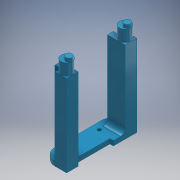
# Autodesk Inventor part: blue_part-july21
Saved by Autodesk Inventor 2017 SP1 (Build 210196100, 196)
## iProperties
Created: 2016-07-25
Part Number: blue_part-july21
Material: Plastique ABS
Document SubType Name: Modeling
Designer: tmonglon
Density: 1.06 g/cm^3
Appearance: Bleu ciel foncé
Author: tmonglon
Autodesk Inventor part; units mm, degrees
ref_plane "YZ Plane" through (0, 0, 0) normal (1, 0, 0) x (0, 1, 0)
ref_plane "XZ Plane" through (0, 0, 0) normal (0, 1, 0) x (-1, 0, 0)
ref_plane "XY Plane" through (0, 0, 0) normal (0, 0, 1) x (1, 0, 0)
sketch "Esquisse1" plane through (0, 0, 0) normal (0, 0, 1) x (1, 0, 0)
  line L0 (0, 0) -> (-10, 0)
  line L1 (-10, 0) -> (-10, 30)
  line L2 (-10, 30) -> (0, 30)
  line L3 (0, 0) -> (-5, 0)
  line L4 (-5, 0) -> (-5, 5)
  line L5 (-5, 5) -> (0, 5)
  line L6 (0, 5) -> (0, 0)
  line L7 (0, 4) -> (-3, 4)
  line L8 (-3, 4) -> (-3, 1)
  line L9 (-3, 1) -> (0, 1)
  line L10 (0, 1) -> (0, 4)
  line L11 (-1.5, 5) -> (-1.5, 20)
  line L12 (-1.5, 20) -> (0, 20)
  line L13 (0, 30) -> (0, 20)
  line L14 (0, 5) -> (0, 0)
  line L15 (0, 29) -> (-3, 29)
  line L16 (-3, 29) -> (-3, 26)
  line L17 (-3, 26) -> (0, 26)
  line L18 (0, 26) -> (0, 29)
  line L19 (0, 25) -> (-5, 25)
  line L20 (-5, 25) -> (-5, 30)
  line L21 (-5, 25) -> (-7.5, 25)
  line L22 (-7.5, 25) -> (-7.5, 27.5)
  line L23 (-7.5, 27.5) -> (-5, 27.5)
  line L24 (-5, 27.5) -> (-5, 25)
  line L25 (-5, 0) -> (-7.5, 0)
  line L26 (-5, 2.5) -> (-5, 0)
  line L27 (-5, 5) -> (-7.5, 5)
  line L28 (-7.5, 5) -> (-7.5, 2.5)
  line L29 (-7.5, 2.5) -> (-5, 2.5)
  line L30 (-5, 2.5) -> (-5, 5)
  line L31 (-3, 26) -> (0, 26)
  line L32 (0, 26) -> (0, 29)
  line L33 (0, 29) -> (-3, 29)
  line L34 (-3, 29) -> (-3, 26)
  line L35 (-3, 1) -> (0, 1)
  line L36 (0, 1) -> (0, 4)
  line L37 (0, 4) -> (-3, 4)
  line L38 (-3, 4) -> (-3, 1)
  dimension "d0" = 10
  dimension "d1" = 30
  dimension "d2" = 5
  dimension "d3" = 5
  dimension "d4" = 3
  dimension "d5" = 3
  dimension "d6" = 1
  dimension "d7" = 15
  dimension "d9" = 3
  dimension "d10" = 3
  dimension "d11" = 1
  dimension "d12" = 5
  dimension "d13" = 5
  dimension "d14" = 2.5
  dimension "d15" = 2.5
  dimension "d20" = 2.5
  dimension "d21" = 2.5
  constraints: 78 end point, 17 parallel, 11 perpendicular, 10 horizontal, 3 point on line, 2 midpoint, 1 vertical
  measures "d0" distance of L0.start L0.end
  measures "d1" distance of L2.end L0.start
  measures "d2" distance of L4.end L5.end
  measures "d3" distance of L3.end L4.end
  measures "d4" distance of L8.end L9.end
  measures "d5" distance of L7.end L8.end
  measures "d6" distance between parallel lines of L5 L7
  measures "d7" distance of L11.start L11.end
  measures "d9" distance of L15.end L16.end
  measures "d10" distance of L16.end L17.end
  measures "d11" distance between parallel lines of L2 L15
  measures "d12" distance of L19.start L19.end
  measures "d13" distance of L19.end L20.end
  measures "d14" distance of L22.end L23.end
  measures "d15" distance of L21.end L22.end
  measures "d20" distance of L28.end L29.end
  measures "d21" distance of L27.end L28.end
extrude "Extrusion1" add sketch "Esquisse1" along normal blind 41.5 contours L0 L4 L5 L6 L7 L8 L9 | L9 L8 L7 L6 | L2 L13 L15 L16 L17 L19 L20 | L13 L17 L16 L15
extrude "Extrusion2" add sketch "Esquisse1" along normal blind 35 contours L29 L28 L27 L4 | L20 L21 L22 L23
extrude "Extrusion4" add sketch "Esquisse1" along normal blind 2 contours L0 L1 L2 L20 L23 L22 L21 L19 L13 L12 L11 L5 L27 L28 L29 L4
fillet "Congé1" radius 5 2 edges at (-10, 0, 1) (-10, 30, 1)
sketch "Esquisse3" plane through (0, 0, 0) normal (0, 0, -1) x (-1, 0, 0)
  circle A0 centre (7, 9) radius 0.7
  circle A1 centre (7, 21) radius 0.7
  line L0 (0, 0) -> (0, 5) projected
  line L1 (0, 20) -> (0, 30) projected
  line L2 (5, 0) -> (0, 0) projected
  dimension "d29" = 1.4
  dimension "d30" = 1.4
  dimension "d31" = 12
  dimension "d32" = 7
  dimension "d33" = 7
  dimension "d34" = 9
  constraints: 2 centre point
  measures "d29" diameter of A0
  measures "d30" diameter of A1
  measures "d31" distance of A1.centre A0.centre
  measures "d32" distance from line of L0 A0.centre
  measures "d33" distance from line of L1 A1.centre
  measures "d34" distance from line of L2 A0.centre
extrude "Extrusion5" cut sketch "Esquisse3" against normal through all
fillet "Congé2" radius 2 2 edges at (-3.75, 25, 2) (-4.5, 5, 2)
sketch "Esquisse8" plane through (0, 0, 41.5) normal (0, 0, 1) x (1, 0, 0)
  line L0 (0, 0) -> (0, 5) projected
  line L1 (0, 5) -> (-5, 5) projected
  line L2 (-5, 5) -> (-5, 0) projected
  line L3 (-5, 0) -> (0, 0) projected
  line L4 (0, 30) -> (-5, 30) projected
  line L5 (-5, 30) -> (-5, 25) projected
  line L6 (-5, 25) -> (0, 25) projected
  line L7 (0, 25) -> (0, 30) projected
  circle A0 centre (-2.5, 2.5) radius 2.4
  circle A1 centre (-2.5, 27.5) radius 2.4
  dimension "d42" = 4.8
  dimension "d43" = 2.5
  dimension "d44" = 2.5
  dimension "d45" = 4.8
  dimension "d48" = 2.5
  dimension "d49" = 2.5
  constraints: 2 centre point
  measures "d42" diameter of A0
  measures "d43" distance from line of L7 A1.centre
  measures "d44" distance from line of L4 A1.centre
  measures "d45" diameter of A1
  measures "d48" distance from line of L0 A0.centre
  measures "d49" distance from line of L3 A0.centre
extrude "Extrusion8" cut sketch "Esquisse8" against normal blind 6.5
sketch "Esquisse9" plane through (-2.5, 2.5, 41.5) normal (0, 0, 1) x (1, 0, 0)
  circle A0 centre (0, 0) radius 2.4 projected
  circle A1 centre (0, 25) radius 2.4 projected
  line L0 (0, 0) -> (3.9146, 0)
  circle A2 centre (1, 0) radius 1.4
  circle A3 centre (0, 0) radius 2.4 projected
  line L1 (0, 25) -> (4.0517, 25)
  circle A4 centre (1, 25) radius 1.4
  point P0 (2.5, -2.5)
  dimension "d52" = 2.8
  dimension "d53" = 2.8
  constraints: 4 end point, 2 centre point, 2 horizontal, 2 point on line, 2 tangent
  measures "d52" diameter of A2
  measures "d53" diameter of A4
extrude "Extrusion9" cut sketch "Esquisse9" against normal blind 1.5
